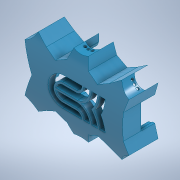
# Autodesk Inventor part: Body1
Saved by Autodesk Inventor 2020 (Build 240168000, 168)
## iProperties
Created: 2019-04-30
Part Number: Body1
Material: Acetal Resin, Black
Document SubType Name: Modeling
Designer: Daniel
Density: 1.425 g/cm^3
Appearance: Sky Blue Dark
Mass: 450.03 g
Surface Area: 768.427 cm^2
Volume: 315.811 cm^3
Author: Daniel
Autodesk Inventor part; units mm, degrees
(part 1 of 6)
ref_plane "YZ Plane" through (0, 0, 0) normal (1, 0, 0) x (0, 1, 0)
sketch "Sketch1" plane through (0, 0, 0) normal (0, 0, 1) x (1, 0, 0)
  circle A0 centre (4.5, -10) radius 1 projected
  circle A1 centre (-4.5, 10) radius 1 projected
  circle A2 centre (4.5, 10) radius 1 projected
  circle A3 centre (-4.5, -10) radius 1 projected
  line L0 (6.2, 11.5) -> (-6.2, 11.5) projected
  line L1 (-6.2, 11.5) -> (-6.2, -11.5) projected
  line L2 (-6.2, -11.5) -> (6.2, -11.5) projected
  line L3 (6.2, -11.5) -> (6.2, 11.5) projected
  arc A4 (1.125, 16.5) -> (0.625, 16) centre (1.125, 16) ccw projected
  line L4 (0.625, 16) -> (0.625, 14.9922) projected
  arc A5 (0.625, 14.9922) -> (0.75, 14.6614) centre (1.125, 14.9922) ccw projected
  arc A6 (-0.75, 14.6614) -> (0.75, 14.6614) centre (0, 14) ccw projected
  arc A7 (-0.75, 14.6614) -> (-0.625, 14.9922) centre (-1.125, 14.9922) ccw projected
  line L5 (-0.625, 14.9922) -> (-0.625, 16) projected
  arc A8 (-0.625, 16) -> (-1.125, 16.5) centre (-1.125, 16) ccw projected
  line L6 (-6.2, 16.5) -> (-1.125, 16.5) projected
  line L7 (-6.2, 16.5) -> (-6.2, 11.5) projected
  line L8 (6.2, 11.5) -> (-6.2, 11.5) projected
  line L9 (6.2, 11.5) -> (6.2, 16.5) projected
  line L10 (1.125, 16.5) -> (6.2, 16.5) projected
  arc A9 (-1.125, -16.5) -> (-0.625, -16) centre (-1.125, -16) ccw projected
  line L11 (-0.625, -16) -> (-0.625, -14.9922) projected
  arc A10 (-0.625, -14.9922) -> (-0.75, -14.6614) centre (-1.125, -14.9922) ccw projected
  arc A11 (0.75, -14.6614) -> (-0.75, -14.6614) centre (0, -14) ccw projected
  arc A12 (0.75, -14.6614) -> (0.625, -14.9922) centre (1.125, -14.9922) ccw projected
  line L12 (0.625, -14.9922) -> (0.625, -16) projected
  arc A13 (0.625, -16) -> (1.125, -16.5) centre (1.125, -16) ccw projected
  line L13 (1.125, -16.5) -> (6.2, -16.5) projected
  line L14 (6.2, -11.5) -> (6.2, -16.5) projected
  line L15 (-6.2, -11.5) -> (6.2, -11.5) projected
  line L16 (-6.2, -16.5) -> (-6.2, -11.5) projected
  line L17 (-6.2, -16.5) -> (-1.125, -16.5) projected
  circle A14 centre (0, -14) radius 1
  circle A15 centre (0, 14) radius 1
  line L18 (6.2, 16.5) -> (-6.2, 16.5)
  line L19 (-6.2, 16.5) -> (-6.2, -16.5)
  line L20 (-6.2, -16.5) -> (6.2, -16.5)
  line L21 (6.2, -16.5) -> (6.2, 16.5)
  line L22 (7, 32) -> (6, 31) projected
  line L23 (7, 32) -> (6, 33) projected
  line L24 (6, 33) -> (-6, 33) projected
  line L25 (-6, 33) -> (-7, 32) projected
  line L26 (-7, 32) -> (-6, 31) projected
  line L27 (-6, 31) -> (6, 31) projected
  line L28 (11.0001, 21.3001) -> (-11.0001, 21.3001)
  line L29 (-11.0001, 21.3001) -> (-11.0001, -21.3001)
  line L30 (-11.0001, -21.3001) -> (11.0001, -21.3001)
  line L31 (11.0001, -21.3001) -> (11.0001, 21.3001)
  arc A16 (11.0001, 21.3001) -> (-11.0001, 21.3001) centre (0, 14) ccw
  circle A17 centre (0, 14) radius 13.202
  line L32 (-13.202, 14) -> (-13.202, -21.3001)
  line L33 (-13.202, -21.3001) -> (-11.0001, -21.3001)
  line L34 (13.202, 14) -> (13.202, -21.3001)
  line L35 (13.202, -21.3001) -> (11.0001, -21.3001)
  line L36 (-13.202, -21.3001) -> (-63.202, -21.3001)
  line L37 (-63.202, -21.3001) -> (-66.3161, -24.4142)
  line L38 (-63.202, -21.3001) -> (-58.798, -21.3001) construction
  line L39 (-66.3161, -24.4142) -> (-81.8724, -39.9705)
  line L40 (-63.202, -21.3001) -> (-88.1629, 3.6608)
  line L41 (-81.8724, -39.9705) -> (-106.8333, -15.0097)
  line L42 (-106.8333, -15.0097) -> (-88.1629, 3.6608)
  arc A18 (-88.1629, 3.6608) -> (-106.8333, -15.0097) centre (-97.4981, -5.6744) ccw
  line L43 (0, 27.202) -> (0, -114)
  line L44 (13.202, -21.3001) -> (63.202, -21.3001)
  line L45 (63.202, -21.3001) -> (66.3161, -24.4142)
  line L46 (63.202, -21.3001) -> (58.798, -21.3001) construction
  line L47 (66.3161, -24.4142) -> (81.8724, -39.9705)
  line L48 (63.202, -21.3001) -> (88.1629, 3.6608)
  line L49 (81.8724, -39.9705) -> (106.8333, -15.0097)
  line L50 (106.8333, -15.0097) -> (88.1629, 3.6608)
  arc A19 (106.8333, -15.0097) -> (88.1629, 3.6608) centre (97.4981, -5.6744) ccw
  line L51 (-38.202, -21.3001) -> (-38.202, -31.3001)
  line L52 (-38.202, -31.3001) -> (-19.202, -21.3001)
  line L53 (-38.202, -31.3001) -> (-57.202, -21.3001)
  line L54 (13.202, -21.3001) -> (19.202, -21.3001)
  line L55 (38.202, -21.3001) -> (38.202, -31.3001)
  line L56 (38.202, -31.3001) -> (19.202, -21.3001)
  line L57 (38.202, -31.3001) -> (57.202, -21.3001)
  line L58 (0, -21.3001) -> (0, -121.3001)
  line L59 (0, -71.3001) -> (81.8724, -71.3001)
  line L60 (81.8724, -71.3001) -> (81.8724, -39.9705)
  line L61 (0, -71.3001) -> (-81.8724, -71.3001)
  line L62 (-81.8724, -71.3001) -> (-81.8724, -39.9705)
  circle A20 centre (4.5, -132.6002) radius 1
  circle A21 centre (-4.5, -152.6002) radius 1
  circle A22 centre (4.5, -152.6002) radius 1
  circle A23 centre (-4.5, -132.6002) radius 1
  line L63 (6.2, -154.1002) -> (-6.2, -154.1002)
  line L64 (-6.2, -154.1002) -> (-6.2, -131.1002)
  line L65 (-6.2, -131.1002) -> (6.2, -131.1002)
  line L66 (6.2, -131.1002) -> (6.2, -154.1002)
  arc A24 (0.625, -158.6002) -> (1.125, -159.1002) centre (1.125, -158.6002) ccw
  line L67 (0.625, -158.6002) -> (0.625, -157.5923)
  arc A25 (0.75, -157.2616) -> (0.625, -157.5923) centre (1.125, -157.5923) ccw
  arc A26 (0.75, -157.2616) -> (-0.75, -157.2616) centre (0, -156.6002) ccw
  arc A27 (-0.625, -157.5923) -> (-0.75, -157.2616) centre (-1.125, -157.5923) ccw
  line L68 (-0.625, -157.5923) -> (-0.625, -158.6002)
  arc A28 (-1.125, -159.1002) -> (-0.625, -158.6002) centre (-1.125, -158.6002) ccw
  line L69 (-6.2, -159.1002) -> (-1.125, -159.1002)
  line L70 (-6.2, -159.1002) -> (-6.2, -154.1002)
  line L71 (6.2, -154.1002) -> (-6.2, -154.1002)
  line L72 (6.2, -154.1002) -> (6.2, -159.1002)
  line L73 (1.125, -159.1002) -> (6.2, -159.1002)
  arc A29 (-0.625, -126.6002) -> (-1.125, -126.1002) centre (-1.125, -126.6002) ccw
  line L74 (-0.625, -126.6002) -> (-0.625, -127.608)
  arc A30 (-0.75, -127.9387) -> (-0.625, -127.608) centre (-1.125, -127.608) ccw
  arc A31 (-0.75, -127.9387) -> (0.75, -127.9387) centre (0, -128.6002) ccw
  arc A32 (0.625, -127.608) -> (0.75, -127.9387) centre (1.125, -127.608) ccw
  line L75 (0.625, -127.608) -> (0.625, -126.6002)
  arc A33 (1.125, -126.1002) -> (0.625, -126.6002) centre (1.125, -126.6002) ccw
  line L76 (1.125, -126.1002) -> (6.2, -126.1002)
  line L77 (6.2, -131.1002) -> (6.2, -126.1002)
  line L78 (-6.2, -131.1002) -> (6.2, -131.1002)
  line L79 (-6.2, -126.1002) -> (-6.2, -131.1002)
  line L80 (-6.2, -126.1002) -> (-1.125, -126.1002)
  circle A34 centre (0, -128.6002) radius 1
  circle A35 centre (0, -156.6002) radius 1
  line L81 (6.2, -159.1002) -> (-6.2, -159.1002)
  line L82 (-6.2, -159.1002) -> (-6.2, -126.1002)
  line L83 (-6.2, -126.1002) -> (6.2, -126.1002)
  line L84 (6.2, -126.1002) -> (6.2, -159.1002)
  line L85 (11.0001, -163.9002) -> (-11.0001, -163.9002)
  line L86 (-11.0001, -163.9002) -> (-11.0001, -121.3001)
  line L87 (-11.0001, -121.3001) -> (11.0001, -121.3001)
  line L88 (11.0001, -121.3001) -> (11.0001, -163.9002)
  arc A36 (-11.0001, -163.9002) -> (11.0001, -163.9002) centre (0, -156.6002) ccw
  circle A37 centre (0, -156.6002) radius 13.202
  line L89 (-13.202, -156.6002) -> (-13.202, -121.3001)
  line L90 (-13.202, -121.3001) -> (-11.0001, -121.3001)
  line L91 (13.202, -156.6002) -> (13.202, -121.3001)
  line L92 (13.202, -121.3001) -> (11.0001, -121.3001)
  line L93 (-13.202, -121.3001) -> (-63.202, -121.3001)
  line L94 (-63.202, -121.3001) -> (-66.3161, -118.186)
  line L95 (-63.202, -121.3001) -> (-58.798, -121.3001) construction
  line L96 (-66.3161, -118.186) -> (-81.8724, -102.6296)
  line L97 (-63.202, -121.3001) -> (-88.1629, -146.2609)
  line L98 (-81.8724, -102.6296) -> (-106.8333, -127.5905)
  line L99 (-106.8333, -127.5905) -> (-88.1629, -146.2609)
  arc A38 (-106.8333, -127.5905) -> (-88.1629, -146.2609) centre (-97.4981, -136.9257) ccw
  line L100 (0, -169.8022) -> (0, -28.6002)
  line L101 (13.202, -121.3001) -> (63.202, -121.3001)
  line L102 (63.202, -121.3001) -> (58.798, -121.3001) construction
  line L103 (63.202, -121.3001) -> (66.3161, -118.186)
  line L104 (66.3161, -118.186) -> (81.8724, -102.6296)
  line L105 (63.202, -121.3001) -> (88.1629, -146.2609)
  line L106 (106.8333, -127.5905) -> (88.1629, -146.2609)
  arc A39 (88.1629, -146.2609) -> (106.8333, -127.5905) centre (97.4981, -136.9257) ccw
  line L107 (81.8724, -102.6296) -> (106.8333, -127.5905)
  line L108 (-38.202, -121.3001) -> (-38.202, -111.3001)
  line L109 (-38.202, -111.3001) -> (-19.202, -121.3001)
  line L110 (-38.202, -111.3001) -> (-57.202, -121.3001)
  line L111 (13.202, -121.3001) -> (19.202, -121.3001)
  line L112 (38.202, -121.3001) -> (38.202, -111.3001)
  line L113 (38.202, -111.3001) -> (19.202, -121.3001)
  line L114 (38.202, -111.3001) -> (57.202, -121.3001)
  line L115 (0, -121.3001) -> (0, -21.3001)
  line L116 (81.8724, -71.3001) -> (81.8724, -102.6296)
  line L117 (-81.8724, -71.3001) -> (-81.8724, -102.6296)
  line L118 (-75.6824, -133.7805) -> (-57.202, -121.3001)
  line L119 (13.202, -138.9501) -> (19.202, -121.3001)
  line L120 (-13.202, -138.9501) -> (-19.202, -121.3001)
  line L121 (-75.6824, -8.8196) -> (-57.202, -21.3001)
  line L122 (-19.202, -21.3001) -> (-13.202, -3.65)
  line L123 (13.202, -3.65) -> (19.202, -21.3001)
  line L124 (57.202, -21.3001) -> (75.6824, -8.8196)
  line L125 (57.202, -121.3001) -> (75.6824, -133.7805)
  line L126 (81.8724, -102.6296) -> (76.663, -73.0854)
  line L127 (81.8724, -102.6296) -> (111.8724, -102.6296) construction
  line L128 (76.663, -73.0854) -> (76.3482, -71.3001)
  line L129 (76.3482, -71.3001) -> (81.8724, -39.9705)
  line L130 (-81.8724, -102.6296) -> (-76.663, -73.0854)
  line L131 (-81.8724, -102.6296) -> (-51.8724, -102.6296) construction
  line L132 (-76.663, -73.0854) -> (-76.3482, -71.3001)
  line L133 (-76.3482, -71.3001) -> (-81.8724, -39.9705)
  line L134 (-94.3529, -27.4901) -> (-76.3482, -71.3001)
  line L135 (-76.3482, -71.3001) -> (-94.3529, -115.1101)
  line L136 (94.3529, -27.4901) -> (81.8724, -71.3001)
  line L137 (81.8724, -71.3001) -> (94.3529, -115.1101)
  circle A40 centre (0, 0) radius 1
  line L138 (63.202, -21.3001) -> (81.8724, -39.9705)
  line L139 (72.5372, -30.6353) -> (75.9313, -27.2412)
  line L140 (75.9313, -27.2412) -> (71.5473, -22.8571)
  line L141 (75.9313, -27.2412) -> (80.3154, -31.6252)
  line L142 (71.5473, -22.8571) -> (94.8818, 0.4774)
  line L143 (94.8818, 0.4774) -> (103.6499, -8.2907)
  line L144 (103.6499, -8.2907) -> (80.3154, -31.6252)
  line L145 (80.3154, -31.6252) -> (71.5473, -22.8571)
  line L146 (75.9313, -27.2412) -> (99.2659, -3.9067)
  line L147 (75.9313, -27.2412) -> (77.6991, -25.4734)
  circle A41 centre (77.6991, -25.4734) radius 1
  line L148 (99.2659, -3.9067) -> (97.4981, -5.6744)
  circle A42 centre (97.4981, -5.6744) radius 1
  circle A43 centre (87.5986, -15.5739) radius 1
  line L149 (97.4981, -136.9257) -> (72.5372, -111.9649)
  line L150 (72.5372, -111.9649) -> (75.9313, -115.359)
  line L151 (75.9313, -115.359) -> (80.3154, -110.9749)
  line L152 (75.9313, -115.359) -> (71.5473, -119.743)
  line L153 (80.3154, -110.9749) -> (103.6499, -134.3094)
  line L154 (103.6499, -134.3094) -> (94.8818, -143.0776)
  line L155 (94.8818, -143.0776) -> (71.5473, -119.743)
  line L156 (71.5473, -119.743) -> (80.3154, -110.9749)
  circle A44 centre (77.6991, -117.1267) radius 1
  line L157 (75.9313, -115.359) -> (77.6991, -117.1267)
  line L158 (97.4981, -136.9257) -> (95.7303, -135.158)
  line L159 (75.9313, -115.359) -> (87.5986, -127.0262)
  circle A45 centre (87.5986, -127.0262) radius 1
  line L160 (-81.8724, -102.6296) -> (-63.202, -121.3001)
  line L161 (-63.202, -121.3001) -> (-72.5372, -111.9649)
  line L162 (-72.5372, -111.9649) -> (-75.9313, -115.359)
  line L163 (-75.9313, -115.359) -> (-80.3154, -110.9749)
  line L164 (-80.3154, -110.9749) -> (-75.9313, -115.359)
  line L165 (-75.9313, -115.359) -> (-71.5473, -119.743)
  line L166 (-71.5473, -119.743) -> (-94.8818, -143.0776)
  line L167 (-94.8818, -143.0776) -> (-103.6499, -134.3094)
  line L168 (-103.6499, -134.3094) -> (-80.3154, -110.9749)
  line L169 (-80.3154, -110.9749) -> (-71.5473, -119.743)
  line L170 (-99.2659, -138.6935) -> (-97.4981, -136.9257)
  circle A46 centre (-97.4981, -136.9257) radius 1
  line L171 (-75.9313, -115.359) -> (-77.6991, -117.1267)
  circle A47 centre (-77.6991, -117.1267) radius 1
  line L172 (-99.2659, -138.6935) -> (-75.9313, -115.359)
  circle A48 centre (-87.5986, -127.0262) radius 1
  line L173 (-81.8724, -39.9705) -> (-63.202, -21.3001)
  line L174 (-81.8724, -39.9705) -> (-72.5372, -30.6353)
  circle A49 centre (0, -142.6002) radius 1
  circle A50 centre (97.4981, -136.9257) radius 1
  line L175 (-81.8724, -39.9705) -> (-63.202, -21.3001)
  line L176 (-63.202, -21.3001) -> (-72.5372, -30.6353)
  line L177 (-72.5372, -30.6353) -> (-75.9313, -27.2412)
  line L178 (-75.9313, -27.2412) -> (-80.3154, -31.6252)
  line L179 (-75.9313, -27.2412) -> (-71.5473, -22.8571)
  line L180 (-80.3154, -31.6252) -> (-103.6499, -8.2907)
  line L181 (-103.6499, -8.2907) -> (-94.8818, 0.4774)
  line L182 (-94.8818, 0.4774) -> (-71.5473, -22.8571)
  line L183 (-71.5473, -22.8571) -> (-80.3154, -31.6252)
  line L184 (-99.2659, -3.9067) -> (-97.4981, -5.6744)
  circle A51 centre (-97.4981, -5.6744) radius 1
  line L185 (-75.9313, -27.2412) -> (-77.6991, -25.4734)
  circle A52 centre (-77.6991, -25.4734) radius 1
  line L186 (-97.4981, -5.6744) -> (-77.6991, -25.4734)
  line L187 (-77.6991, -25.4734) -> (-87.5986, -15.5739)
  circle A53 centre (-87.5986, -15.5739) radius 1
  point P0 (-11.0001, 21.3001)
  dimension "d0" = 50
  dimension "d1" = 4.404
  dimension "d2" = 135
  dimension "d3" = 22
  dimension "d4" = 35.3
  dimension "d5" = 35.3
  dimension "d6" = 98.2878
  dimension "d7" = 10
  dimension "d8" = 19
  dimension "d9" = 19
  dimension "d10" = 6
  dimension "d11" = 10
  dimension "d12" = 19
  dimension "d13" = 100
  dimension "d14" = 30
  dimension "d15" = 100
  dimension "d16" = 30
  dimension "d17" = 80
  dimension "d18" = 2
  dimension "d19" = 4.8
  dimension "d20" = 6.2
  dimension "d21" = 6.2
  dimension "d22" = 33
  dimension "d23" = 2.5
  dimension "d24" = 2
  dimension "d25" = 2.5
  dimension "d26" = 2
  dimension "d27" = 2
  dimension "d28" = 90
  dimension "d29" = 6.2
  dimension "d30" = 6.2
  dimension "d31" = 33
  dimension "d32" = 2
  dimension "d33" = 2.5
  dimension "d35" = 2
  dimension "d36" = 4.8
  dimension "d37" = 6.2
  dimension "d38" = 6.2
  dimension "d39" = 33
  dimension "d40" = 2.5
  dimension "d41" = 2
  dimension "d42" = 2.5
  dimension "d43" = 2
  dimension "d44" = 2
  dimension "d45" = 2.5
  dimension "d46" = 19.402
  dimension "d47" = 169.4403
  dimension "d48" = 155.4403
  dimension "d58" = 2
  dimension "d59" = 2
  dimension "d71" = 4.8
  dimension "d72" = 33
  dimension "d73" = 2.5
  dimension "d74" = 2
  dimension "d75" = 2.5
  dimension "d76" = 2
  dimension "d77" = 14
  dimension "d78" = 2
  dimension "d79" = 106.7312
  dimension "d80" = 94.3312
  constraints: 328 end point, 86 symmetric about line, 40 centre point, 39 point on circle, 26 midpoint, 24 point on line, 23 perpendicular, 19 coincident, 16 parallel, 7 horizontal, 5 collinear, 4 equal radius, 4 tangent, 4 vertical, 3 equal length, 24 other
  measures "d0" distance of L32.end L36.end
  measures "d1" distance of L36.end L37.end
  measures "d2" angle of L37 L38
  measures "d3" distance of L37.end L39.end
  measures "d4" distance of L36.end L40.end
  measures "d5" distance of L39.end L41.end
  measures "d6" distance from line of L43.end L22
  measures "d7" distance of L51.start L51.end
  measures "d8" horizontal distance of L51.end L52.end
  measures "d9" horizontal distance of L51.end L53.end
  measures "d10" distance of L34.end L54.end
  measures "d11" distance of L55.start L55.end
  measures "d12" horizontal distance of L55.end L57.end
  measures "d13" distance of L58.start L58.end
  measures "d14" distance of L104.end L126.end
  measures "d15" angle of L127 L126
  measures "d16" distance of L117.end L130.end
  measures "d17" angle of L131 L130
  measures "d18" diameter of A40
  measures "d19" distance of L139.start L139.end
  measures "d20" distance of L139.end L140.end
  measures "d21" distance of L139.end L141.end
  measures "d22" distance of L140.end L142.end
  measures "d23" distance of L139.end L147.end
  measures "d24" diameter of A41
  measures "d25" distance of L146.end L148.end
  measures "d26" diameter of A42
  measures "d27" diameter of A43
  measures "d28" angle of L22 L141
  measures "d29" distance of L150.end L151.end
  measures "d30" distance of L150.end L152.end
  measures "d31" distance of L151.end L153.end
  measures "d32" diameter of A44
  measures "d33" distance of L149.start L158.end
  measures "d35" diameter of A45
  measures "d36" distance of L161.end L162.end
  measures "d37" distance of L162.end L163.end
  measures "d38" distance of L162.end L165.end
  measures "d39" distance of L165.end L166.end
  measures "d40" distance of L170.start L170.end
  measures "d41" diameter of A46
  measures "d42" distance of L162.end L171.end
  measures "d43" diameter of A47
  measures "d44" diameter of A48
  measures "d45" distance between parallel lines of L106 L154
  measures "d46" distance between parallel lines of L155 L107
  measures "d47" distance from line of L159.end L22
  measures "d48" distance from line of L157.end L22
  measures "d58" diameter of A49
  measures "d59" diameter of A50
  measures "d71" distance of L174.end L177.end
  measures "d72" distance of L178.end L180.end
  measures "d73" distance of L184.start L184.end
  measures "d74" diameter of A51
  measures "d75" distance of L177.end L185.end
  measures "d76" diameter of A52
  measures "d77" distance of L186.end L187.end
  measures "d78" diameter of A53
  measures "d79" distance between parallel lines of L23 L180
  measures "d80" distance from line of L179.end L23
extrude "Extrusion1" add sketch "Sketch1" along normal blind 10 contours L9 L10 L18 L43 L28 L31 A17 L3 | A17 L31 L30 L43 L20 L13 L14 L3 | L1 A17 L29 L28 L43 L18 L6 L7 | A17 L34 L35 L31 | L31 A17 | L1 L16 L17 L20 L43 L30 L29 A17 | L35 L44 L56 L57 L45 L47 L129 L59 L43 L30 | L28 L43 A16 | A17 L29 | L29 L33 L32 A17 | L43 L61 L133 L39 L37 L36 L53 L52 L33 L30 | L34 L123 L44 | L28 A16 L43 | L36 L122 L32 | L59 L128 L126 L104 L103 L101 L114 L113 L92 L87 L58 L43 | L43 L58 L87 L90 L93 L109 L110 L94 L96 L130 L132 L61 | L129 L60 L59 | L59 L116 L126 L128 | L134 L62 L133 | L132 L130 L117 L135 | L124 L48 L44 | L100 L83 L80 L79 L64 A37 L86 L87 | L87 L88 A37 L66 L77 L76 L83 L100 | L137 L107 L116 | L60 L49 L136 | L47 L139 L141 L144 L50 L49 | L41 L42 L180 L178 L177 L39 | L62 L134 L41 | L117 L98 L135 | L48 L50 L142 L140 L139 L47 L45 | L36 L40 L121 | L86 A37 L89 L90 | L92 L91 A37 L88 | L107 L106 L153 L151 L149 L104 | L96 L162 L163 L168 L99 L98 | L177 L179 L182 L42 L40 L37 L39 | A19 L50 L144 L143 L142 | A37 L64 L70 L69 L81 L100 L85 L86 | L86 A37 | L89 L120 L93 | A37 L88 | L88 L85 L100 L81 L73 L72 L66 A37 | L101 L119 L91 | L149 L152 L155 L106 L105 L103 L104 | A39 L106 L155 L154 L153 | L96 L94 L97 L99 L166 L165 L162 | A18 L42 L182 L181 L180 | L99 L168 L167 L166 A38 | L85 L100 A36 | A36 L100 L85 | L105 L125 L101 | L93 L118 L97
sketch "Sketch2" plane through (0, 0, 0) normal (0, 0, -1) x (-1, 0, 0)
  arc A0 (-1.125, -16.5) -> (-0.625, -16) centre (-1.125, -16) ccw projected
  line L0 (-0.625, -16) -> (-0.625, -14.9922) projected
  arc A1 (-0.625, -14.9922) -> (-0.75, -14.6614) centre (-1.125, -14.9922) ccw projected
  arc A2 (0.75, -14.6614) -> (-0.75, -14.6614) centre (0, -14) ccw projected
  arc A3 (0.75, -14.6614) -> (0.625, -14.9922) centre (1.125, -14.9922) ccw projected
  line L1 (0.625, -14.9922) -> (0.625, -16) projected
  arc A4 (0.625, -16) -> (1.125, -16.5) centre (1.125, -16) ccw projected
  line L2 (1.125, -16.5) -> (6.2, -16.5) projected
  line L3 (6.2, -11.5) -> (6.2, -16.5) projected
  line L4 (-6.2, -11.5) -> (6.2, -11.5) projected
  line L5 (-6.2, -16.5) -> (-6.2, -11.5) projected
  line L6 (-6.2, -16.5) -> (-1.125, -16.5) projected
  arc A5 (1.125, 16.5) -> (0.625, 16) centre (1.125, 16) ccw projected
  line L7 (0.625, 16) -> (0.625, 14.9922) projected
  arc A6 (0.625, 14.9922) -> (0.75, 14.6614) centre (1.125, 14.9922) ccw projected
  arc A7 (-0.75, 14.6614) -> (0.75, 14.6614) centre (0, 14) ccw projected
  arc A8 (-0.75, 14.6614) -> (-0.625, 14.9922) centre (-1.125, 14.9922) ccw projected
  line L8 (-0.625, 14.9922) -> (-0.625, 16) projected
  arc A9 (-0.625, 16) -> (-1.125, 16.5) centre (-1.125, 16) ccw projected
  line L9 (-6.2, 16.5) -> (-1.125, 16.5) projected
  line L10 (-6.2, 16.5) -> (-6.2, 11.5) projected
  line L11 (6.2, 11.5) -> (-6.2, 11.5) projected
  line L12 (6.2, 11.5) -> (6.2, 16.5) projected
  line L13 (1.125, 16.5) -> (6.2, 16.5) projected
  arc A10 (-76.7268, -28.0367) -> (-76.7268, -27.3296) centre (-77.0804, -27.6831) ccw projected
  line L14 (-76.7268, -27.3296) -> (-77.4395, -26.6169) projected
  arc A11 (-77.4395, -26.6169) -> (-77.7617, -26.4715) centre (-77.793, -26.9705) ccw projected
  arc A12 (-76.7011, -25.4108) -> (-77.7617, -26.4715) centre (-77.6991, -25.4734) ccw projected
  arc A13 (-76.7011, -25.4108) -> (-76.5556, -25.733) centre (-76.202, -25.3795) ccw projected
  line L15 (-76.5556, -25.733) -> (-75.8429, -26.4457) projected
  arc A14 (-75.8429, -26.4457) -> (-75.1358, -26.4457) centre (-75.4894, -26.0921) ccw projected
  line L16 (-75.1358, -26.4457) -> (-71.5473, -22.8571) projected
  line L17 (-75.0828, -19.3216) -> (-71.5473, -22.8571) projected
  line L18 (-83.8509, -28.0897) -> (-75.0828, -19.3216) projected
  line L19 (-80.3154, -31.6252) -> (-83.8509, -28.0897) projected
  line L20 (-80.3154, -31.6252) -> (-76.7268, -28.0367) projected
  arc A15 (-98.4704, -3.1112) -> (-98.4704, -3.8183) centre (-98.1168, -3.4647) ccw projected
  line L21 (-98.4704, -3.8183) -> (-97.7577, -4.5309) projected
  arc A16 (-97.7577, -4.5309) -> (-97.4355, -4.6764) centre (-97.4042, -4.1774) ccw projected
  arc A17 (-98.4961, -5.7371) -> (-97.4355, -4.6764) centre (-97.4981, -5.6744) ccw projected
  arc A18 (-98.4961, -5.7371) -> (-98.6416, -5.4148) centre (-98.9951, -5.7684) ccw projected
  line L22 (-98.6416, -5.4148) -> (-99.3542, -4.7022) projected
  arc A19 (-99.3542, -4.7022) -> (-100.0614, -4.7022) centre (-99.7078, -5.0557) ccw projected
  line L23 (-103.6499, -8.2907) -> (-100.0614, -4.7022) projected
  line L24 (-103.6499, -8.2907) -> (-100.1144, -11.8263) projected
  line L25 (-91.3463, -3.0581) -> (-100.1144, -11.8263) projected
  line L26 (-91.3463, -3.0581) -> (-94.8818, 0.4774) projected
  line L27 (-98.4704, -3.1112) -> (-94.8818, 0.4774) projected
  arc A20 (-75.1358, -116.1545) -> (-75.8429, -116.1545) centre (-75.4894, -116.508) ccw projected
  line L28 (-75.8429, -116.1545) -> (-76.5556, -116.8671) projected
  arc A21 (-76.5556, -116.8671) -> (-76.7011, -117.1894) centre (-76.202, -117.2207) ccw projected
  arc A22 (-77.7617, -116.1287) -> (-76.7011, -117.1894) centre (-77.6991, -117.1267) ccw projected
  arc A23 (-77.7617, -116.1287) -> (-77.4395, -115.9832) centre (-77.793, -115.6297) ccw projected
  line L29 (-77.4395, -115.9832) -> (-76.7268, -115.2706) projected
  arc A24 (-76.7268, -115.2706) -> (-76.7268, -114.5635) centre (-77.0804, -114.917) ccw projected
  line L30 (-76.7268, -114.5635) -> (-80.3154, -110.9749) projected
  line L31 (-83.8509, -114.5104) -> (-80.3154, -110.9749) projected
  line L32 (-75.0828, -123.2786) -> (-83.8509, -114.5104) projected
  line L33 (-71.5473, -119.743) -> (-75.0828, -123.2786) projected
  line L34 (-71.5473, -119.743) -> (-75.1358, -116.1545) projected
  arc A25 (-100.0614, -137.898) -> (-99.3542, -137.898) centre (-99.7078, -137.5444) ccw projected
  line L35 (-99.3542, -137.898) -> (-98.6416, -137.1853) projected
  arc A26 (-98.6416, -137.1853) -> (-98.4961, -136.8631) centre (-98.9951, -136.8318) ccw projected
  arc A27 (-97.4355, -137.9238) -> (-98.4961, -136.8631) centre (-97.4981, -136.9257) ccw projected
  arc A28 (-97.4355, -137.9238) -> (-97.7577, -138.0692) centre (-97.4042, -138.4228) ccw projected
  line L36 (-97.7577, -138.0692) -> (-98.4704, -138.7819) projected
  arc A29 (-98.4704, -138.7819) -> (-98.4704, -139.489) centre (-98.1168, -139.1354) ccw projected
  line L37 (-94.8818, -143.0776) -> (-98.4704, -139.489) projected
  line L38 (-94.8818, -143.0776) -> (-91.3463, -139.542) projected
  line L39 (-100.1144, -130.7739) -> (-91.3463, -139.542) projected
  line L40 (-100.1144, -130.7739) -> (-103.6499, -134.3094) projected
  line L41 (-100.0614, -137.898) -> (-103.6499, -134.3094) projected
  arc A30 (1.125, -126.1002) -> (0.625, -126.6002) centre (1.125, -126.6002) ccw projected
  line L42 (0.625, -126.6002) -> (0.625, -127.608) projected
  arc A31 (0.625, -127.608) -> (0.75, -127.9387) centre (1.125, -127.608) ccw projected
  arc A32 (-0.75, -127.9387) -> (0.75, -127.9387) centre (0, -128.6002) ccw projected
  arc A33 (-0.75, -127.9387) -> (-0.625, -127.608) centre (-1.125, -127.608) ccw projected
  line L43 (-0.625, -127.608) -> (-0.625, -126.6002) projected
  arc A34 (-0.625, -126.6002) -> (-1.125, -126.1002) centre (-1.125, -126.6002) ccw projected
  line L44 (-1.125, -126.1002) -> (-6.2, -126.1002) projected
  line L45 (-6.2, -131.1002) -> (-6.2, -126.1002) projected
  line L46 (6.2, -131.1002) -> (-6.2, -131.1002) projected
  line L47 (6.2, -126.1002) -> (6.2, -131.1002) projected
  line L48 (6.2, -126.1002) -> (1.125, -126.1002) projected
  arc A35 (-1.125, -159.1002) -> (-0.625, -158.6002) centre (-1.125, -158.6002) ccw projected
  line L49 (-0.625, -158.6002) -> (-0.625, -157.5923) projected
  arc A36 (-0.625, -157.5923) -> (-0.75, -157.2616) centre (-1.125, -157.5923) ccw projected
  arc A37 (0.75, -157.2616) -> (-0.75, -157.2616) centre (0, -156.6002) ccw projected
  arc A38 (0.75, -157.2616) -> (0.625, -157.5923) centre (1.125, -157.5923) ccw projected
  line L50 (0.625, -157.5923) -> (0.625, -158.6002) projected
  arc A39 (0.625, -158.6002) -> (1.125, -159.1002) centre (1.125, -158.6002) ccw projected
  line L51 (6.2, -159.1002) -> (1.125, -159.1002) projected
  line L52 (6.2, -159.1002) -> (6.2, -154.1002) projected
  line L53 (-6.2, -154.1002) -> (6.2, -154.1002) projected
  line L54 (-6.2, -154.1002) -> (-6.2, -159.1002) projected
  line L55 (-1.125, -159.1002) -> (-6.2, -159.1002) projected
  arc A40 (76.7268, -114.5635) -> (76.7268, -115.2706) centre (77.0804, -114.917) ccw projected
  line L56 (76.7268, -115.2706) -> (77.4395, -115.9832) projected
  arc A41 (77.4395, -115.9832) -> (77.7617, -116.1287) centre (77.793, -115.6297) ccw projected
  arc A42 (76.7011, -117.1894) -> (77.7617, -116.1287) centre (77.6991, -117.1267) ccw projected
  arc A43 (76.7011, -117.1894) -> (76.5556, -116.8671) centre (76.202, -117.2207) ccw projected
  line L57 (76.5556, -116.8671) -> (75.8429, -116.1545) projected
  arc A44 (75.8429, -116.1545) -> (75.1358, -116.1545) centre (75.4894, -116.508) ccw projected
  line L58 (75.1358, -116.1545) -> (71.5473, -119.743) projected
  line L59 (75.0828, -123.2786) -> (71.5473, -119.743) projected
  line L60 (83.8509, -114.5104) -> (75.0828, -123.2786) projected
  line L61 (80.3154, -110.9749) -> (83.8509, -114.5104) projected
  line L62 (80.3154, -110.9749) -> (76.7268, -114.5635) projected
  arc A45 (98.4704, -139.489) -> (98.4704, -138.7819) centre (98.1168, -139.1354) ccw projected
  line L63 (98.4704, -138.7819) -> (97.7577, -138.0692) projected
  arc A46 (97.7577, -138.0692) -> (97.4355, -137.9238) centre (97.4042, -138.4228) ccw projected
  arc A47 (98.4961, -136.8631) -> (97.4355, -137.9238) centre (97.4981, -136.9257) ccw projected
  arc A48 (98.4961, -136.8631) -> (98.6416, -137.1853) centre (98.9951, -136.8318) ccw projected
  line L64 (98.6416, -137.1853) -> (99.3542, -137.898) projected
  arc A49 (99.3542, -137.898) -> (100.0614, -137.898) centre (99.7078, -137.5444) ccw projected
  line L65 (103.6499, -134.3094) -> (100.0614, -137.898) projected
  line L66 (103.6499, -134.3094) -> (100.1144, -130.7739) projected
  line L67 (91.3463, -139.542) -> (100.1144, -130.7739) projected
  line L68 (91.3463, -139.542) -> (94.8818, -143.0776) projected
  line L69 (98.4704, -139.489) -> (94.8818, -143.0776) projected
  arc A50 (100.0614, -4.7022) -> (99.3542, -4.7022) centre (99.7078, -5.0557) ccw projected
  line L70 (99.3542, -4.7022) -> (98.6416, -5.4148) projected
  arc A51 (98.6416, -5.4148) -> (98.4961, -5.7371) centre (98.9951, -5.7684) ccw projected
  arc A52 (97.4355, -4.6764) -> (98.4961, -5.7371) centre (97.4981, -5.6744) ccw projected
  arc A53 (97.4355, -4.6764) -> (97.7577, -4.5309) centre (97.4042, -4.1774) ccw projected
  line L71 (97.7577, -4.5309) -> (98.4704, -3.8183) projected
  arc A54 (98.4704, -3.8183) -> (98.4704, -3.1112) centre (98.1168, -3.4647) ccw projected
  line L72 (94.8818, 0.4774) -> (98.4704, -3.1112) projected
  line L73 (94.8818, 0.4774) -> (91.3463, -3.0581) projected
  line L74 (100.1144, -11.8263) -> (91.3463, -3.0581) projected
  line L75 (100.1144, -11.8263) -> (103.6499, -8.2907) projected
  line L76 (100.0614, -4.7022) -> (103.6499, -8.2907) projected
  arc A55 (75.1358, -26.4457) -> (75.8429, -26.4457) centre (75.4894, -26.0921) ccw projected
  line L77 (75.8429, -26.4457) -> (76.5556, -25.733) projected
  arc A56 (76.5556, -25.733) -> (76.7011, -25.4108) centre (76.202, -25.3795) ccw projected
  arc A57 (77.7617, -26.4715) -> (76.7011, -25.4108) centre (77.6991, -25.4734) ccw projected
  arc A58 (77.7617, -26.4715) -> (77.4395, -26.6169) centre (77.793, -26.9705) ccw projected
  line L78 (77.4395, -26.6169) -> (76.7268, -27.3296) projected
  arc A59 (76.7268, -27.3296) -> (76.7268, -28.0367) centre (77.0804, -27.6831) ccw projected
  line L79 (76.7268, -28.0367) -> (80.3154, -31.6252) projected
  line L80 (83.8509, -28.0897) -> (80.3154, -31.6252) projected
  line L81 (75.0828, -19.3216) -> (83.8509, -28.0897) projected
  line L82 (71.5473, -22.8571) -> (75.0828, -19.3216) projected
  line L83 (71.5473, -22.8571) -> (75.1358, -26.4457) projected
  line L84 (-103.6499, -134.3094) -> (-94.8818, -143.0776) projected
  line L85 (-94.8818, -143.0776) -> (-91.3463, -139.542)
  line L86 (-91.3463, -139.542) -> (-100.1144, -130.7739)
  line L87 (-100.1144, -130.7739) -> (-103.6499, -134.3094)
  line L88 (-103.6499, -134.3094) -> (-94.8818, -143.0776)
  line L89 (-94.8818, -143.0776) -> (-71.5473, -119.743) projected
  line L90 (-75.0828, -123.2786) -> (-83.8509, -114.5104)
  line L91 (-83.8509, -114.5104) -> (-80.3154, -110.9749)
  line L92 (-80.3154, -110.9749) -> (-71.5473, -119.743)
  line L93 (-71.5473, -119.743) -> (-75.0828, -123.2786)
  line L94 (-80.3154, -31.6252) -> (-71.5473, -22.8571) projected
  line L95 (-71.5473, -22.8571) -> (-80.3154, -31.6252)
  line L96 (-80.3154, -31.6252) -> (-83.8509, -28.0897)
  line L97 (-83.8509, -28.0897) -> (-75.0828, -19.3216)
  line L98 (-75.0828, -19.3216) -> (-71.5473, -22.8571)
  line L99 (-91.3463, -3.0581) -> (-100.1144, -11.8263)
  line L100 (-100.1144, -11.8263) -> (-103.6499, -8.2907)
  line L101 (-103.6499, -8.2907) -> (-94.8818, 0.4774)
  line L102 (-94.8818, 0.4774) -> (-91.3463, -3.0581)
  line L103 (-6.2, -16.5) -> (6.2, -16.5) projected
  line L104 (6.2, -16.5) -> (-6.2, -16.5)
  line L105 (-6.2, -16.5) -> (-6.2, -11.5)
  line L106 (-6.2, -11.5) -> (6.2, -11.5)
  line L107 (6.2, -11.5) -> (6.2, -16.5)
  line L108 (-6.2, 11.5) -> (6.2, 11.5)
  line L109 (6.2, 11.5) -> (6.2, 16.5)
  line L110 (6.2, 16.5) -> (-6.2, 16.5)
  line L111 (-6.2, 16.5) -> (-6.2, 11.5)
  line L112 (100.1144, -11.8263) -> (91.3463, -3.0581)
  line L113 (91.3463, -3.0581) -> (94.8818, 0.4774)
  line L114 (94.8818, 0.4774) -> (103.6499, -8.2907)
  line L115 (103.6499, -8.2907) -> (100.1144, -11.8263)
  line L116 (75.0828, -19.3216) -> (83.8509, -28.0897)
  line L117 (83.8509, -28.0897) -> (80.3154, -31.6252)
  line L118 (80.3154, -31.6252) -> (71.5473, -22.8571)
  line L119 (71.5473, -22.8571) -> (75.0828, -19.3216)
  line L120 (80.3154, -110.9749) -> (71.5473, -119.743) projected
  line L121 (80.3154, -110.9749) -> (83.8509, -114.5104)
  line L122 (83.8509, -114.5104) -> (75.0828, -123.2786)
  line L123 (75.0828, -123.2786) -> (71.5473, -119.743)
  line L124 (71.5473, -119.743) -> (80.3154, -110.9749)
  line L125 (103.6499, -134.3094) -> (80.3154, -110.9749) projected
  line L126 (100.1144, -130.7739) -> (103.6499, -134.3094)
  line L127 (103.6499, -134.3094) -> (94.8818, -143.0776)
  line L128 (94.8818, -143.0776) -> (91.3463, -139.542)
  line L129 (91.3463, -139.542) -> (100.1144, -130.7739)
  line L130 (6.2, -126.1002) -> (-6.2, -126.1002) projected
  line L131 (6.2, -126.1002) -> (-6.2, -126.1002)
  line L132 (-6.2, -126.1002) -> (-6.2, -131.1002)
  line L133 (-6.2, -131.1002) -> (6.2, -131.1002)
  line L134 (6.2, -131.1002) -> (6.2, -126.1002)
  line L135 (6.2, -154.1002) -> (-6.2, -154.1002)
  line L136 (-6.2, -154.1002) -> (-6.2, -159.1002)
  line L137 (-6.2, -159.1002) -> (6.2, -159.1002)
  line L138 (6.2, -159.1002) -> (6.2, -154.1002)
  point P0 (0, 0)
  point P1 (-98.4704, -3.1112)
  point P2 (-100.0614, -4.7022)
  point P3 (1.125, 16.5)
  point P4 (-1.125, 16.5)
  point P5 (98.4704, -3.1112)
  point P6 (1.125, 16.5)
  point P7 (-1.125, 16.5)
  point P8 (-1.125, -159.1002)
  point P9 (1.125, -159.1002)
  point P10 (6.2, -159.1002)
  point P11 (-6.2, -159.1002)
  point P12 (-100.0614, -4.7022)
  point P13 (-98.4704, -3.1112)
  point P14 (-94.8818, 0.4774)
  point P15 (-103.6499, -8.2907)
  dimension "d83" = 146.5831
  dimension "d84" = 113.5831
  dimension "d85" = 207.6918
  dimension "d86" = 235.6918
  dimension "d87" = 89.1087
  dimension "d88" = 12.4
  dimension "d89" = 56.1087
  dimension "d90" = 12.4
  dimension "d91" = 23
  dimension "d92" = 142.6002
  dimension "d93" = 170.6002
  dimension "d94" = 142.6002
  constraints: 96 end point, 24 parallel, 15 perpendicular, 8 collinear
  measures "d83" distance between parallel lines of L65 L87
  measures "d84" distance between parallel lines of L66 L92
  measures "d85" distance between parallel lines of L65 L97
  measures "d86" distance between parallel lines of L65 L101
  measures "d87" distance between parallel lines of L125 L114
  measures "d88" distance between parallel lines of L125 L128
  measures "d89" distance between parallel lines of L66 L118
  measures "d90" distance between parallel lines of L66 L123
  measures "d91" distance between parallel lines of L11 L106
  measures "d92" distance between parallel lines of L11 L133
  measures "d93" distance between parallel lines of L11 L137
  measures "d94" distance between parallel lines of L48 L110
extrude "Extrusion2" add sketch "Sketch2" against normal blind 19
sketch "Sketch3" plane through (0, 0, 0) normal (0, 0, -1) x (-1, 0, 0)
  line L0 (13.202, 14) -> (13.202, -3.65) projected
  arc A0 (13.202, 14) -> (-13.202, 14) centre (0, 14) ccw projected
  line L1 (-13.202, -3.65) -> (-13.202, 14) projected
  line L2 (-19.202, -21.3001) -> (-13.202, -3.65) projected
  line L3 (-38.202, -31.3001) -> (-19.202, -21.3001) projected
  line L4 (-57.202, -21.3001) -> (-38.202, -31.3001) projected
  line L5 (-75.6824, -8.8196) -> (-57.202, -21.3001) projected
  line L6 (-88.1629, 3.6608) -> (-75.6824, -8.8196) projected
  arc A1 (-88.1629, 3.6608) -> (-106.8333, -15.0097) centre (-97.4981, -5.6744) ccw projected
  line L7 (-94.3529, -27.4901) -> (-106.8333, -15.0097) projected
  line L8 (-81.8724, -71.3001) -> (-94.3529, -27.4901) projected
  line L9 (-94.3529, -115.1101) -> (-81.8724, -71.3001) projected
  line L10 (-106.8333, -127.5905) -> (-94.3529, -115.1101) projected
  arc A2 (-106.8333, -127.5905) -> (-88.1629, -146.2609) centre (-97.4981, -136.9257) ccw projected
  line L11 (-75.6824, -133.7805) -> (-88.1629, -146.2609) projected
  line L12 (-57.202, -121.3001) -> (-75.6824, -133.7805) projected
  line L13 (-38.202, -111.3001) -> (-57.202, -121.3001) projected
  line L14 (-19.202, -121.3001) -> (-38.202, -111.3001) projected
  line L15 (-13.202, -138.9501) -> (-19.202, -121.3001) projected
  line L16 (-13.202, -156.6002) -> (-13.202, -138.9501) projected
  arc A3 (-13.202, -156.6002) -> (13.202, -156.6002) centre (0, -156.6002) ccw projected
  line L17 (13.202, -138.9501) -> (13.202, -156.6002) projected
  line L18 (19.202, -121.3001) -> (13.202, -138.9501) projected
  line L19 (38.202, -111.3001) -> (19.202, -121.3001) projected
  line L20 (57.202, -121.3001) -> (38.202, -111.3001) projected
  line L21 (75.6824, -133.7805) -> (57.202, -121.3001) projected
  line L22 (88.1629, -146.2609) -> (75.6824, -133.7805) projected
  arc A4 (88.1629, -146.2609) -> (106.8333, -127.5905) centre (97.4981, -136.9257) ccw projected
  line L23 (94.3529, -115.1101) -> (106.8333, -127.5905) projected
  line L24 (76.3482, -71.3001) -> (94.3529, -115.1101) projected
  line L25 (94.3529, -27.4901) -> (76.3482, -71.3001) projected
  line L26 (106.8333, -15.0097) -> (94.3529, -27.4901) projected
  arc A5 (106.8333, -15.0097) -> (88.1629, 3.6608) centre (97.4981, -5.6744) ccw projected
  line L27 (75.6824, -8.8196) -> (88.1629, 3.6608) projected
  line L28 (38.202, -31.3001) -> (57.202, -21.3001) projected
  line L29 (19.202, -21.3001) -> (38.202, -31.3001) projected
  line L30 (13.202, -3.65) -> (19.202, -21.3001) projected
  line L31 (-6.2, 11.5) -> (-6.2, -11.5) projected
  line L32 (6.2, -11.5) -> (6.2, 11.5) projected
  line L33 (6.2, -154.1002) -> (6.2, -131.1002) projected
  line L34 (-6.2, -131.1002) -> (-6.2, -154.1002) projected
  line L35 (-100.1144, -11.8263) -> (-83.8509, -28.0897) projected
  line L36 (-75.0828, -19.3216) -> (-91.3463, -3.0581) projected
  line L37 (75.0828, -123.2786) -> (91.3463, -139.542) projected
  line L38 (100.1144, -130.7739) -> (83.8509, -114.5104) projected
  line L39 (83.8509, -28.0897) -> (100.1144, -11.8263) projected
  line L40 (91.3463, -3.0581) -> (75.0828, -19.3216) projected
  line L41 (-91.3463, -139.542) -> (-75.0828, -123.2786) projected
  line L42 (-83.8509, -114.5104) -> (-100.1144, -130.7739) projected
  line L43 (13.202, 14) -> (13.202, -3.65) projected
  arc A6 (13.202, 14) -> (-13.202, 14) centre (0, 14) ccw projected
  line L44 (-13.202, -3.65) -> (-13.202, 14) projected
  line L45 (-19.202, -21.3001) -> (-13.202, -3.65) projected
  line L46 (-38.202, -31.3001) -> (-19.202, -21.3001) projected
  line L47 (-57.202, -21.3001) -> (-38.202, -31.3001) projected
  line L48 (-75.6824, -8.8196) -> (-57.202, -21.3001) projected
  line L49 (-88.1629, 3.6608) -> (-75.6824, -8.8196) projected
  arc A7 (-88.1629, 3.6608) -> (-106.8333, -15.0097) centre (-97.4981, -5.6744) ccw projected
  line L50 (-94.3529, -27.4901) -> (-106.8333, -15.0097) projected
  line L51 (-81.8724, -71.3001) -> (-94.3529, -27.4901) projected
  line L52 (-94.3529, -115.1101) -> (-81.8724, -71.3001) projected
  line L53 (-106.8333, -127.5905) -> (-94.3529, -115.1101) projected
  arc A8 (-106.8333, -127.5905) -> (-88.1629, -146.2609) centre (-97.4981, -136.9257) ccw projected
  line L54 (-75.6824, -133.7805) -> (-88.1629, -146.2609) projected
  line L55 (-57.202, -121.3001) -> (-75.6824, -133.7805) projected
  line L56 (-38.202, -111.3001) -> (-57.202, -121.3001) projected
  line L57 (-19.202, -121.3001) -> (-38.202, -111.3001) projected
  line L58 (-13.202, -138.9501) -> (-19.202, -121.3001) projected
  line L59 (-13.202, -156.6002) -> (-13.202, -138.9501) projected
  arc A9 (-13.202, -156.6002) -> (13.202, -156.6002) centre (0, -156.6002) ccw projected
  line L60 (13.202, -138.9501) -> (13.202, -156.6002) projected
  line L61 (19.202, -121.3001) -> (13.202, -138.9501) projected
  line L62 (38.202, -111.3001) -> (19.202, -121.3001) projected
  line L63 (57.202, -121.3001) -> (38.202, -111.3001) projected
  line L64 (75.6824, -133.7805) -> (57.202, -121.3001) projected
  line L65 (88.1629, -146.2609) -> (75.6824, -133.7805) projected
  arc A10 (88.1629, -146.2609) -> (106.8333, -127.5905) centre (97.4981, -136.9257) ccw projected
  line L66 (94.3529, -115.1101) -> (106.8333, -127.5905) projected
  line L67 (76.3482, -71.3001) -> (94.3529, -115.1101) projected
  line L68 (94.3529, -27.4901) -> (76.3482, -71.3001) projected
  line L69 (106.8333, -15.0097) -> (94.3529, -27.4901) projected
  arc A11 (106.8333, -15.0097) -> (88.1629, 3.6608) centre (97.4981, -5.6744) ccw projected
  line L70 (75.6824, -8.8196) -> (88.1629, 3.6608) projected
  line L71 (38.202, -31.3001) -> (57.202, -21.3001) projected
  line L72 (19.202, -21.3001) -> (38.202, -31.3001) projected
  line L73 (13.202, -3.65) -> (19.202, -21.3001) projected
  line L74 (-6.2, 11.5) -> (-6.2, -11.5) projected
  line L75 (6.2, -11.5) -> (6.2, 11.5) projected
  line L76 (6.2, -154.1002) -> (6.2, -131.1002) projected
  line L77 (-6.2, -131.1002) -> (-6.2, -154.1002) projected
  line L78 (-100.1144, -11.8263) -> (-83.8509, -28.0897) projected
  line L79 (-75.0828, -19.3216) -> (-91.3463, -3.0581) projected
  line L80 (75.0828, -123.2786) -> (91.3463, -139.542) projected
  line L81 (100.1144, -130.7739) -> (83.8509, -114.5104) projected
  line L82 (83.8509, -28.0897) -> (100.1144, -11.8263) projected
  line L83 (91.3463, -3.0581) -> (75.0828, -19.3216) projected
  line L84 (-91.3463, -139.542) -> (-75.0828, -123.2786) projected
  line L85 (-83.8509, -114.5104) -> (-100.1144, -130.7739) projected
  line L86 (57.202, -21.3001) -> (75.6824, -8.8196) projected
  line L87 (57.202, -21.3001) -> (75.6824, -8.8196) projected
  line L88 (6.2, -11.5) -> (-6.2, -11.5) projected
  line L89 (-6.2, 11.5) -> (6.2, 11.5) projected
  line L90 (6.2, -154.1002) -> (-6.2, -154.1002) projected
  line L91 (-6.2, -131.1002) -> (6.2, -131.1002) projected
  line L92 (-75.0828, -19.3216) -> (-83.8509, -28.0897) projected
  line L93 (-100.1144, -11.8263) -> (-91.3463, -3.0581) projected
  line L94 (100.1144, -130.7739) -> (91.3463, -139.542) projected
  line L95 (75.0828, -123.2786) -> (83.8509, -114.5104) projected
  line L96 (91.3463, -3.0581) -> (100.1144, -11.8263) projected
  line L97 (83.8509, -28.0897) -> (75.0828, -19.3216) projected
  line L98 (-83.8509, -114.5104) -> (-75.0828, -123.2786) projected
  line L99 (-91.3463, -139.542) -> (-100.1144, -130.7739) projected
  line L100 (6.2, -11.5) -> (-6.2, -11.5) projected
  line L101 (-6.2, 11.5) -> (6.2, 11.5) projected
  line L102 (6.2, -154.1002) -> (-6.2, -154.1002) projected
  line L103 (-6.2, -131.1002) -> (6.2, -131.1002) projected
  line L104 (-75.0828, -19.3216) -> (-83.8509, -28.0897) projected
  line L105 (-100.1144, -11.8263) -> (-91.3463, -3.0581) projected
  line L106 (100.1144, -130.7739) -> (91.3463, -139.542) projected
  line L107 (75.0828, -123.2786) -> (83.8509, -114.5104) projected
  line L108 (91.3463, -3.0581) -> (100.1144, -11.8263) projected
  line L109 (83.8509, -28.0897) -> (75.0828, -19.3216) projected
  line L110 (-83.8509, -114.5104) -> (-75.0828, -123.2786) projected
  line L111 (-91.3463, -139.542) -> (-100.1144, -130.7739) projected
  point P0 (0, 0)
extrude "Extrusion3" add sketch "Sketch3" along normal blind 5 contours L0 L30 L29 L28 L86 L27 A5 L26 L25 L24 L23 A4 L22 L21 L20 L19 L18 L17 A3 L16 L15 L14 L13 L12 L11 A2 L10 L9 L8 L7 A1 L6 L5 L4 L3 L2 L1 A0 | L89 L32 L88 L31 | L90 L34 L91 L33 | L93 L36 L92 L35 | L95 L38 L94 L37 | L97 L40 L96 L39 | L99 L42 L98 L41
sketch "Sketch6" plane through (0, 0, -5) normal (0, 0, -1) x (-1, 0, 0)
  circle A0 centre (0, -148.1002) radius 0.6 projected
  circle A1 centre (91.4877, -130.9153) radius 0.6 projected
  circle A2 centre (91.4877, -11.6848) radius 0.6 projected
  circle A3 centre (0, 5.5) radius 0.7 projected
  circle A4 centre (-91.4877, -11.6848) radius 0.6 projected
  circle A5 centre (-91.4877, -130.9153) radius 0.6 projected
  point P0 (0, 0)
hole "Hole2" at (-91.4877, -11.6848, -5) at (-91.4877, -130.9153, -5) at (0, -148.1002, -5) at (91.4877, -130.9153, -5) at (91.4877, -11.6848, -5) at (0, 5.5, -5) direction (0, 0, 1) diameter 10 depth 3.8
sketch "Sketch13" plane through (0, 0, 10) normal (0, 0, 1) x (1, 0, 0)
  line L0 (81.8724, -71.3001) -> (94.3529, -27.4901) projected
  line L1 (81.8724, -71.3001) -> (76.8724, -71.3001)
  line L2 (76.8724, -71.3001) -> (76.8724, -93.8001)
  line L3 (76.8724, -93.8001) -> (76.8724, -48.8001)
  line L4 (76.8724, -48.8001) -> (88.2822, -48.8001)
  line L5 (81.8724, -71.3001) -> (88.2822, -48.8001)
  line L6 (76.8724, -93.8001) -> (88.2822, -93.8001)
  line L7 (94.3529, -115.1101) -> (81.8724, -71.3001) projected
  line L8 (88.2822, -93.8001) -> (81.8724, -71.3001)
  dimension "d207" = 5
  dimension "d208" = 22.5
  dimension "d209" = 45
  constraints: 14 end point, 3 point on line, 2 horizontal, 2 perpendicular
  measures "d207" distance of L0.start L1.end
  measures "d208" distance of L1.end L2.end
  measures "d209" distance of L2.end L3.end
extrude "Extrusion10" add sketch "Sketch13" along normal blind 25
sketch "Sketch16" plane through (76.8724, -93.8001, 10) normal (-1, 0, 0) x (0, 0, 1)
  line L0 (25, 0) -> (25, 22.5)
  line L1 (0, -21.31) -> (0, 0)
  line L2 (25, 0) -> (0, 0)
  line L3 (0, 45) -> (25, 45)
  line L4 (25, 0) -> (0, 0)
  line L5 (0, 0) -> (0, 45)
  line L6 (0, 45) -> (25, 45)
  line L7 (25, 45) -> (25, 0)
  line L8 (0, 45) -> (2.5, 45)
  line L9 (0, 0) -> (25, 0)
  line L10 (2.5, 45) -> (22.5, 45)
  line L11 (22.5, 45) -> (22.5, 0)
  line L12 (22.5, 0) -> (2.5, 0)
  line L13 (2.5, 0) -> (2.5, 45)
  line L14 (2.5, 45) -> (2.5, 36)
  line L15 (2.5, 36) -> (12.5, 36)
  circle A0 centre (12.5, 36) radius 8
  line L16 (12.5, 36) -> (12.5, 9)
  circle A1 centre (12.5, 9) radius 8
  circle A2 centre (12.5, 36) radius 8.3
  circle A3 centre (12.5, 9) radius 8.3
  line L17 (2.5, 45) -> (2.5, 43.5)
  line L18 (2.5, 43.5) -> (4, 43.5)
  circle A4 centre (4, 43.5) radius 1
  line L19 (25, 45) -> (23.5, 45)
  line L20 (23.5, 45) -> (23.5, 43.5)
  circle A5 centre (23.5, 43.5) radius 1
  line L21 (25, 0) -> (23.5, 0)
  line L22 (23.5, 0) -> (23.5, 1.5)
  circle A6 centre (23.5, 1.5) radius 1
  line L23 (2.5, 0) -> (2.5, 1.5)
  line L24 (2.5, 1.5) -> (4, 1.5)
  circle A7 centre (4, 1.5) radius 1
  line L25 (24.5, 43.5) -> (24.5, 1.5)
  line L26 (12.5, 27.7) -> (24.5, 27.7)
  line L27 (22.5, 27.7) -> (22.5, 17.2)
  line L28 (22.5, 27.7) -> (22.5, 25.95)
  line L29 (22.5, 25.95) -> (19, 25.95)
  line L30 (22.5, 25.95) -> (26, 25.95) construction
  line L31 (22.5, 25.95) -> (22.5, 18.95)
  line L32 (22.5, 18.95) -> (19, 18.95)
  line L33 (19, 18.95) -> (19, 25.95)
  arc A8 (22.5, 25.95) -> (19, 25.95) centre (20.75, 25.95) ccw
  arc A9 (19, 18.95) -> (22.5, 18.95) centre (20.75, 18.95) ccw
  arc A10 (22.8, 25.95) -> (18.7, 25.95) centre (20.75, 25.95) ccw
  line L34 (18.7, 18.95) -> (18.7, 25.95)
  line L35 (22.8, 25.95) -> (22.8, 18.95)
  arc A11 (18.7, 18.95) -> (22.8, 18.95) centre (20.75, 18.95) ccw
  line L36 (22.5, 43.5) -> (21.5, 43.5)
  circle A12 centre (21.5, 43.45) radius 1
  circle A13 centre (21.5, 1.45) radius 1
  circle A14 centre (4.5, 1.45) radius 1
  circle A15 centre (4.5, 43.45) radius 1
  arc A16 (2.5, 18.95) -> (6, 18.95) centre (4.25, 18.95) ccw
  arc A17 (2.2, 18.95) -> (6.3, 18.95) centre (4.25, 18.95) ccw
  line L37 (2.5, 18.95) -> (6, 18.95)
  line L38 (6, 18.95) -> (6, 25.95)
  line L39 (6.3, 18.95) -> (6.3, 25.95)
  line L40 (2.5, 25.95) -> (6, 25.95)
  arc A18 (6, 25.95) -> (2.5, 25.95) centre (4.25, 25.95) ccw
  arc A19 (6.3, 25.95) -> (2.2, 25.95) centre (4.25, 25.95) ccw
  line L41 (2.2, 25.95) -> (2.2, 18.95)
  point P0 (-10, 93.8001)
  point P1 (-10, 93.8001)
  point P2 (18.7, 25.95)
  point P3 (18.7, 18.95)
  point P4 (2.2, 25.95)
  point P5 (6.3, 18.95)
  dimension "d270" = 2
  dimension "d253" = 2.5
  dimension "d254" = 20
  dimension "d255" = 9
  dimension "d256" = 10
  dimension "d257" = 16
  dimension "d258" = 27
  dimension "d259" = 16
  dimension "d260" = 0.3
  dimension "d261" = 0.3
  dimension "d262" = 1.5
  dimension "d263" = 1.5
  dimension "d264" = 2
  dimension "d265" = 1.5
  dimension "d266" = 1.5
  dimension "d267" = 2
  dimension "d268" = 1.5
  dimension "d269" = 1.5
  dimension "d271" = 1.5
  dimension "d272" = 1.5
  dimension "d273" = 2
  dimension "d274" = 10.5
  dimension "d275" = 1.75
  dimension "d276" = 3.5
  dimension "d277" = 180
  dimension "d278" = 7
  dimension "d279" = 0.3
  dimension "d280" = 0.3
  dimension "d281" = 0.3
  dimension "d282" = 0.3
  dimension "d283" = 1
  constraints: 84 end point, 18 centre point, 18 point on circle, 16 point on line, 14 symmetric about line, 9 perpendicular, 8 parallel, 6 coincident, 5 horizontal, 5 tangent, 2 vertical, 1 collinear, 1 horizontal alignment, 1 vertical alignment, 16 other
  measures "d253" distance of L3.start L8.end
  measures "d254" distance of L11.end L12.end
  measures "d255" distance of L8.end L14.end
  measures "d256" distance of L14.end L15.end
  measures "d257" diameter of A0
  measures "d258" distance of L16.start L16.end
  measures "d259" diameter of A1
  measures "d261" radial gap between concentric circles of A3 A1
  measures "d262" distance of L8.end L17.end
  measures "d263" distance of L17.end L18.end
  measures "d264" diameter of A4
  measures "d265" distance of L6.end L19.end
  measures "d266" distance of L19.end L20.end
  measures "d267" diameter of A5
  measures "d268" distance of L0.start L21.end
  measures "d269" distance of L21.end L22.end
  measures "d271" distance of L12.end L23.end
  measures "d272" distance of L23.end L24.end
  measures "d273" diameter of A7
  measures "d274" distance of L27.start L27.end
  measures "d275" distance of L27.start L28.end
  measures "d276" distance of L28.end L29.end
  measures "d277" angle of L29 L30
  measures "d278" distance of L28.end L31.end
  measures "d279" distance between parallel lines of L35 L31
  measures "d280" radial gap between concentric circles of A10 A8
  measures "d281" distance between parallel lines of L33 L34
  measures "d282" radial gap between concentric circles of A11 A9
  measures "d283" distance of L36.start L36.end
extrude "Extrusion15" cut sketch "Sketch16" against normal blind 4.3 contours A17 L41 A19 L13 | L13 A16 L38 A18 A19 L39 A17 | L37 A16 | L13 L40 L38 L37 | A18 L40